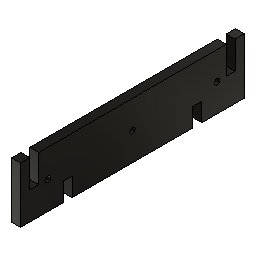
CameraHolder v3 (Autodesk Fusion 360 design; units mm, degrees)
Autodesk Fusion 360 part; units mm, degrees
sketch "Sketch1" plane through (0, 0, 0) normal (1, 0, 0) x (0, 1, 0)
  line L0 (-60.2, 30) -> (-60.2, 0)
  line L1 (-60.2, 0) -> (-37.3, 0)
  line L2 (-37.3, 0) -> (-37.3, 10)
  line L3 (-37.3, 10) -> (-32.5, 10)
  line L4 (-32.5, 10) -> (-32.5, 0)
  line L5 (-32.5, 0) -> (32.5, 0)
  line L6 (32.5, 0) -> (32.5, 10)
  line L7 (32.5, 10) -> (37.3, 10)
  line L8 (37.3, 10) -> (37.3, 0)
  line L9 (37.3, 0) -> (60.2, 0)
  line L10 (60.2, 0) -> (60.2, 30)
  line L11 (60.2, 30) -> (55.2, 30)
  line L12 (55.2, 30) -> (55.2, 15)
  line L13 (55.2, 15) -> (50.4, 15)
  line L14 (50.4, 15) -> (50.4, 30)
  line L15 (50.4, 30) -> (-50.4, 30)
  line L16 (-50.4, 30) -> (-50.4, 15)
  line L17 (-50.4, 15) -> (-55.2, 15)
  line L18 (-55.2, 15) -> (-55.2, 30)
  line L19 (-55.2, 30) -> (-60.2, 30)
  line L20 (-55.2, 30) -> (-50.4, 30) construction
  line L21 (50.4, 30) -> (55.2, 30) construction
  line L22 (37.3, 0) -> (32.5, 0) construction
  line L23 (-32.5, 0) -> (-37.3, 0) construction
  line L24 (-50.4, 15) -> (50.4, 15) construction
  line L25 (0, 0) -> (0, 15) construction
  line L26 (0, 15) -> (0, 30) construction
  circle A0 centre (0, 15) radius 1.5
  circle A1 centre (-45.4, 15) radius 1.5
  circle A2 centre (45.4, 15) radius 1.5
  line L27 (-32.5, 10) -> (32.5, 10) construction
  point P0 (0, 15)
  point P1 (0, 15)
  point P2 (0, 30)
  dimension "d1" = 4.8
  dimension "d2" = 4.8
  dimension "d3" = 4.8
  dimension "d4" = 4.8
  dimension "d7" = 15
  dimension "d9" = 30
  dimension "d10" = 65
  dimension "d11" = 120.4
  dimension "d12" = 100.8
  dimension "d13" = 5
  dimension "d14" = 3
  dimension "d15" = 3
  dimension "d16" = 5
  dimension "d17" = 3
  dimension "d18" = 5
  dimension "d21" = 10
  constraint vertical L0
  constraint perpendicular L0 L1
  constraint perpendicular L1 L2
  constraint perpendicular L0 L3
  constraint perpendicular L1 L4
  constraint perpendicular L4 L5
  constraint perpendicular L3 L6
  constraint perpendicular L6 L7
  constraint perpendicular L7 L8
  constraint perpendicular L8 L9
  constraint perpendicular L9 L10
  constraint perpendicular L0 L11
  constraint perpendicular L11 L12
  constraint perpendicular L0 L13
  constraint perpendicular L13 L14
  constraint perpendicular L14 L15
  constraint perpendicular L15 L16
  constraint perpendicular L16 L17
  constraint perpendicular L15 L18
  constraint perpendicular L0 L19
  constraint perpendicular L18 L20
  constraint perpendicular L12 L21
  constraint perpendicular L6 L22
  constraint perpendicular L2 L23
  constraint perpendicular L14 L24
  constraint midpoint L24 P1
  constraint midpoint L5 L25.start
  constraint midpoint L15 P2
  constraint coincident L25.start origin
  constraint coincident P1 P0
  constraint coincident P2 L26.end
  constraint coincident L24 A1.centre
  constraint coincident L24 A2.centre
  constraint perpendicular L24 L25
  constraint perpendicular L6 L27
  measures "d1" distance of L2 L4
  measures "d2" distance of L6 L8
  measures "d3" distance of L12 L14
  measures "d4" distance of L16 L18
  measures "d7" distance of L15 L24
  measures "d9" distance of L0.start L0.end
  measures "d10" distance of L4 L6
  measures "d11" distance of L0 L10
  measures "d12" distance of L14 L16
  measures "d13" distance of L10 L12
  measures "d14" diameter of A0
  measures "d15" diameter of A1
  measures "d16" distance of L16 A1.centre
  measures "d17" diameter of A2
  measures "d18" distance of L14 A2.centre
  measures "d21" distance of L3 L5
extrude "Extrude1" add sketch "Sketch1" along normal blind 4.8
